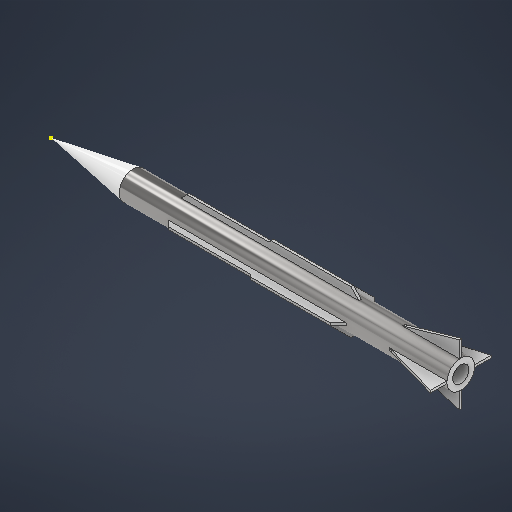
# Autodesk Inventor part: idk
Saved by Autodesk Inventor 2026.3 (Build 303398000, 398)
## iProperties
Created: 2026-04-13
Part Number: idk
Material: Genérico
Document SubType Name: Modeling
Designer: warri
Density: 1 g/cm^3
Appearance: Padrão
Author: warri
Autodesk Inventor part; units mm, degrees
ref_plane "YZ Plane" through (0, 0, 0) normal (1, 0, 0) x (0, 1, 0)
ref_plane "XZ Plane" through (0, 0, 0) normal (0, 1, 0) x (-1, 0, 0)
ref_plane "XY Plane" through (0, 0, 0) normal (0, 0, 1) x (1, 0, 0)
sketch "Esboço2" plane through (0, 0, 0) normal (0, 0, 1) x (1, 0, 0)
  line L0 (0, 0) -> (250, 0)
  line L1 (0, 0) -> (50, 8.5)
  line L2 (0, 0) -> (50.7174, 0) construction
  line L3 (50, 8.5) -> (250, 8.5)
  line L4 (250, 8.5) -> (250, 0)
  line L5 (50, 8.5) -> (50, 0)
  line L6 (50, 8.5) -> (60, 8.5)
  line L7 (60, 8.5) -> (60, 0)
  line L8 (250, 0) -> (369.4937, 0)
  dimension "d5" = 17
  dimension "d7" = 50
  dimension "d9" = 10
  dimension "d61" = 200
  constraints: 18 end point, 4 horizontal, 3 point on line, 2 perpendicular, 1 equal length, 1 vertical
  measures "d5" diameter of L3 L0
  measures "d7" horizontal distance of L1.end L0.start
  measures "d9" distance of L1.end L6.end
  measures "d61" distance of L1.end L3.end
revolve "Revolução1" add sketch "Esboço2" angle 360 about axis through (0, 0, 0) along (1, 0, 0)
sketch "Esboço3" plane through (0, 0, 0) normal (0, 0, 1) x (1, 0, 0)
  line L0 (50, -8.5) -> (250, -8.5) projected
  line L1 (50, -8.5) -> (80, -8.5)
  line L2 (80, -8.5) -> (83.5355, -12.0355)
  line L3 (80, -8.5) -> (85, -8.5) construction
  line L4 (83.5355, -12.0355) -> (133.5355, -12.0355)
  line L5 (133.5355, -12.0355) -> (133.5355, -8.5)
  line L6 (133.5355, -12.0355) -> (134.9497, -13.4497)
  line L7 (134.9497, -13.4497) -> (183.6612, -13.4497)
  line L8 (183.6612, -13.4497) -> (183.6612, -8.5)
  line L9 (183.6612, -13.4497) -> (185.6612, -13.4497) construction
  line L10 (50, -8.5) -> (250, -8.5) projected
  line L11 (183.6612, -13.4497) -> (188.6109, -8.5)
  point P0 (0, 0)
  dimension "d11" = 30
  dimension "d12" = 5
  dimension "d13" = 45
  dimension "d14" = 50
  dimension "d15" = 2
  constraints: 20 end point, 4 horizontal, 4 point on line, 2 perpendicular, 1 equal length
  measures "d11" distance of L0.start L1.end
  measures "d12" distance of L1.end L2.end
  measures "d13" angle of L2 L3
  measures "d14" distance of L2.end L4.end
  measures "d15" distance of L4.end L6.end
extrude "Extrusão1" add sketch "Esboço3" along normal mid plane 1.5
pattern_circular "Padrão circular1" count 4 over 360 about axis through (150, 0, 0) along (1, 0, 0) of "Extrusão1"
sketch "Esboço5" plane through (0, 0, 0) normal (0, 1, 0) x (-1, 0, 0)
  line L0 (-80, -8.5) -> (-188.6109, -8.5) projected
  line L1 (-50, -8.5) -> (-250, -8.5) projected
  line L2 (-250, 8.5) -> (-250, -8.5) projected
  line L3 (-250, -8.5) -> (-250, -18.5)
  line L4 (-250, -18.5) -> (-215, -8.5)
  point P0 (0, 0)
  point P1 (-183.6612, -8.5)
  point P2 (-185.4738, -8.5)
  dimension "d46" = 10
  dimension "d62" = 35
  constraints: 4 end point, 1 point on line, 1 vertical
  measures "d46" distance of L1.end L3.end
  measures "d62" horizontal distance of L3.end L4.end
sketch "Esboço7" plane through (250, 0, 0) normal (1, 0, 0) x (0, -1, 0)
  circle A0 centre (0, 0) radius 5
  dimension "d38" = 10
  constraints: 1 centre point, 1 coincident
  measures "d38" diameter of A0
hole "Furo1" at (250, 0, 0) direction (-1, 0, 0) diameter 10 depth 8 tip angle 118
extrude "Extrusão5" add sketch "Esboço5" along normal mid plane 1.5
pattern_circular "Padrão circular5" count 4 over 360 about axis through (150, 0, 0) along (1, 0, 0) of "Extrusão5"
sketch "Esboço10" plane through (0, 0, 0) normal (0, 0, 1) x (1, 0, 0)
  point P0 (0, 0)
